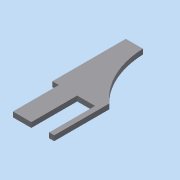
# Autodesk Inventor part: brazos
Saved by Autodesk Inventor 2015 (Build 190159000, 159)
## iProperties
Created: 2017-10-02
Part Number: brazos
Material: Generic
Document SubType Name: Modeling
Designer: macbook
Density: 1 g/cm^3
Appearance: Default
Author: macbook
Autodesk Inventor part; units mm, degrees
ref_plane "YZ Plane" through (0, 0, 0) normal (1, 0, 0) x (0, 1, 0)
ref_plane "XZ Plane" through (0, 0, 0) normal (0, 1, 0) x (-1, 0, 0)
ref_plane "XY Plane" through (0, 0, 0) normal (0, 0, 1) x (1, 0, 0)
sketch "Sketch1" plane through (0, 0, 0) normal (0, 0, 1) x (1, 0, 0)
  line L0 (46.5, 0) -> (46.5, -50)
  line L1 (46.5, -50) -> (52, -50)
  line L2 (52, -50) -> (52, 0)
  line L3 (46.5, 0) -> (27.071, 0)
  line L4 (27.071, 0) -> (27.071, -50)
  line L5 (27.071, -50) -> (7.071, -50)
  line L6 (7.071, -50) -> (7.071, 0)
  line L7 (0, 0) -> (7.071, 0)
  line L8 (0, 80) -> (0, 0)
  arc A0 (18.6268, 80) -> (52, 10) centre (115.8042, 83.3748) ccw
  line L9 (0, 80) -> (18.6268, 80)
  line L10 (52, 10) -> (52, 0)
  dimension "d12" = 5.5
  dimension "d13" = 19.429
  dimension "d14" = 20
  dimension "d15" = 50
  dimension "d21" = 80
  constraints: 22 end point, 3 horizontal, 3 perpendicular, 2 point on circle, 2 vertical, 1 centre point, 1 parallel, 1 point on line
  measures "d12" distance of L2.start L0.end
  measures "d13" distance of L3.start L3.end
  measures "d14" distance of L5.start L6.start
  measures "d15" distance between parallel lines of L1 L3
  measures "d21" distance of point (0, 0) L8.start
extrude "Extrusion2" add sketch "Sketch1" along normal blind 5.5
body "Solid2"
